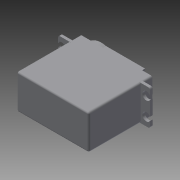
# Autodesk Inventor part: servo
Saved by Autodesk Inventor 2015 SP2 (Build 190223200, 223)
## iProperties
Created: 2016-09-01
Part Number: servo
Material: Generic
Document SubType Name: Modeling
Designer: jm799
Density: 1 g/cm^3
Appearance: Default
Author: jm799
Autodesk Inventor part; units mm, degrees
ref_plane "XZ Plane" through (0, 0, 0) normal (0, 1, 0) x (-1, 0, 0)
ref_plane "XY Plane" through (0, 0, 0) normal (0, 0, 1) x (1, 0, 0)
sketch "Sketch4" plane through (0, 0, 0) normal (0, 1, 0) x (-1, 0, 0)
  line L0 (21.5786, 9.75) -> (-18.7214, 9.75)
  line L1 (-18.7214, 9.75) -> (-18.7214, -9.75)
  line L2 (-18.7214, -9.75) -> (21.5786, -9.75)
  line L3 (21.5786, -9.75) -> (21.5786, 9.75)
  point P0 (0, 0)
  point P1 (21.5786, 0)
  dimension "d6" = 19.5
  dimension "d7" = 40.3
  constraints: 8 end point, 2 parallel, 1 horizontal, 1 horizontal alignment, 1 midpoint, 1 perpendicular
  measures "d6" distance of L0.end L1.end
  measures "d7" distance of L1.end L2.end
extrude "Extrusion2" add sketch "Sketch4" along normal blind 35.5
sketch "Sketch5" plane through (0, 35.5, 0) normal (0, 1, 0) x (1, 0, 0)
  point P0 (0, 0)
sketch "Sketch6" plane through (0, 35.5, 0) normal (0, 1, 0) x (1, 0, 0)
  point P0 (0, 0)
sketch "Sketch7" plane through (0, 35.5, 0) normal (0, 1, 0) x (1, 0, 0)
  point P0 (0, 0)
sketch "Sketch9" plane through (0, 35.5, 0) normal (0, 1, 0) x (1, 0, 0)
  circle A0 centre (-11.7806, 0) radius 9.75
  line L0 (18.7214, 9.75) -> (-21.5786, 9.75) projected
  point P0 (0, 0)
  constraints: 1 centre point, 1 tangent
extrude "Extrusion3" add sketch "Sketch9" along normal blind 2
sketch "Sketch12" plane through (0, 35.5, 0) normal (0, 1, 0) x (1, 0, 0)
  arc A0 (-11.7806, -9.75) -> (-11.7806, 9.75) centre (-11.7806, 0) ccw projected
  arc A1 (-9.1237, -9.381) -> (-9.0416, 9.3574) centre (-11.7806, 0) ccw
  line L0 (-9.1237, -9.381) -> (12.6403, -9.381)
  line L1 (12.6403, -9.381) -> (12.6403, 9.3574)
  line L2 (12.6403, 9.3574) -> (-9.0416, 9.3574)
  point P0 (0, 0)
  constraints: 6 end point, 4 point on circle, 2 perpendicular, 1 centre point, 1 concentric, 1 horizontal
extrude "Extrusion4" add sketch "Sketch12" along normal blind 2
sketch "Sketch13" plane through (0, 35.5, 0) normal (0, 1, 0) x (1, 0, 0)
  line L0 (-21.5786, 9.75) -> (-21.5786, -9.75) construction
  line L1 (-21.5786, 0) -> (18, 0) construction
  line L2 (12.6403, -9.381) -> (12.6403, 9.3574) projected
  arc A0 (12.6403, -6) -> (15.5036, 0) centre (8.5831, -0.3807) ccw
  arc A1 (15.5036, 0) -> (12.6403, 6) centre (8.5831, 0.3807) ccw
  line L3 (12.6403, -6) -> (12.6403, 6)
  line L4 (12.6403, 9.3574) -> (12.6403, -9.381) projected
  point P0 (0, 0)
  constraints: 4 end point, 4 point on circle, 2 centre point, 2 point on line, 2 symmetric about line, 1 collinear, 1 horizontal, 1 midpoint, 1 other
extrude "Extrusion5" add sketch "Sketch13" along normal blind 1.8
sketch "Sketch14" plane through (0, 37.5, 0) normal (0, 1, 0) x (1, 0, 0)
  arc A0 (-9.0416, 9.3574) -> (-9.1237, -9.381) centre (-11.7806, 0) ccw projected
  circle A1 centre (-11.7806, 0) radius 6.395
  point P0 (0, 0)
  dimension "d16" = 12.79
  constraints: 1 centre point, 1 coincident
  measures "d16" diameter of A1
extrude "Extrusion6" add sketch "Sketch14" along normal blind 1.2
sketch "Sketch16" plane through (-11.7806, 38.7, 0) normal (0, 1, 0) x (1, 0, 0)
  circle A0 centre (0, 0) radius 6.395 projected
  circle A1 centre (0, 0) radius 5.6569
  point P0 (11.7806, 0)
  constraints: 1 centre point, 1 coincident
extrude "Extrusion7" add sketch "Sketch16" along normal blind 0.6 contours A1
sketch "Sketch17" plane through (-11.7806, 39.3, 0) normal (0, 1, 0) x (1, 0, 0)
  circle A0 centre (0, 0) radius 6.395 projected
  circle A1 centre (0, 0) radius 2.85
  point P0 (11.7806, 0)
  dimension "d21" = 5.7
  constraints: 1 centre point, 1 coincident
  measures "d21" diameter of A1
extrude "Extrusion8" add sketch "Sketch17" along normal blind 3 contours A1
sketch "Sketch18" plane through (-11.7806, 42.3, 0) normal (0, 1, 0) x (1, 0, 0)
  circle A0 centre (0, 0) radius 2.85 projected
  circle A1 centre (0, 0) radius 1.4142
  point P0 (11.7806, 0)
  constraints: 1 centre point, 1 coincident
extrude "Extrusion9" cut sketch "Sketch18" against normal blind 3 contours A1
sketch "Sketch19" plane through (-21.5786, 0, -9.75) normal (-1, 0, 0) x (0, 0, 1)
  line L0 (0, 35.5) -> (0, 30.5) construction
  line L1 (19.5, 0) -> (19.5, 35.5) projected
  line L2 (0, 30.5) -> (19.5, 30.5)
  line L3 (19.5, 30.5) -> (19.5, 29)
  line L4 (19.5, 29) -> (0, 29)
  line L5 (0, 29) -> (0, 30.5)
  point P0 (9.75, 0)
  dimension "d26" = 5
  constraints: 10 end point, 2 parallel, 1 horizontal, 1 perpendicular, 1 point on line, 1 vertical
  measures "d26" distance of L0.start L0.end
extrude "Extrusion10" add sketch "Sketch19" along normal blind 5.8
sketch "Sketch20" plane through (-21.5786, 30.5, 9.75) normal (0, 1, 0) x (1, 0, 0)
  point P0 (21.5786, 9.75)
sketch "Sketch22" plane through (-21.5786, 30.5, 9.75) normal (0, 1, 0) x (1, 0, 0)
  circle A0 centre (-3.8003, 4.6866) radius 2.25
  line L0 (-11.4938, 9.75) -> (0.0481, 9.75) construction
  arc A1 (9.7981, 19.5) -> (9.7981, 0) centre (9.7981, 9.75) ccw construction
  circle A2 centre (-3.8003, 14.8134) radius 2.25
  point P0 (21.5786, 9.75)
  dimension "d29" = 4.5
  constraints: 2 centre point, 2 end point, 1 horizontal, 1 point on circle
  measures "d29" diameter of A0
hole "Hole1" at (-25.3789, 30.5, 5.0634) at (-25.3789, 30.5, -5.0634) direction (0, -1, 0) diameter 4.5 depth 8 tip angle 118
fillet "Fillet1" radius 1 1 edges at (-27.3786, 29.75, 9.75)
fillet "Fillet2" radius 1 1 edges at (-27.3786, 29.75, -9.75)
fillet "Fillet3" radius 1 4 edges at (-21.5786, 33, 9.75) (-21.5786, 33, -9.75) (18.7214, 17.75, 9.75) (18.7214, 17.75, -9.75)
fillet "Fillet4" radius 1 2 edges at (-21.5786, 14.5, 9.75) (-21.5786, 14.5, -9.75)
ref_plane "Work Plane4" through (-1.75, 0, 0) normal (1, 0, 0) x (0, 1, 0)
mirror "Mirror2" about plane through (-1.75, 0, 0) normal (1, 0, 0) of "Extrusion10", "Hole1", "Fillet1", "Fillet2"
fillet "Fillet5" radius 1 8 edges at (-1.4286, 0, 9.75) (18.4285, 0, 9.4571) (18.7214, 0, 0) (18.4285, 0, -9.4571) (-1.4286, 0, -9.75) (-21.2858, 0, -9.4571) (-21.5786, 0, 0) (-21.2858, 0, 9.4571)
sketch "Sketch26" plane through (0, 35.5, 0) normal (0, 1, 0) x (1, 0, 0)
  point P0 (0, 0)
body "Solid2"
